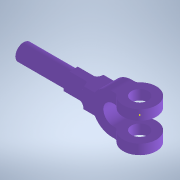
# Autodesk Inventor part: Fork end
Saved by Autodesk Inventor 2021 (Build 250183000, 183)
## iProperties
Created: 2020-01-29
Part Number: Fork end
Material: Plástico PC/ABS
Document SubType Name: Modeling
Designer: aidan
Density: 0.357273 g/cm^3
Appearance: Suave - Blanco
Author: aidan
Autodesk Inventor part; units mm, degrees
ref_plane "YZ Plane" through (0, 0, 0) normal (1, 0, 0) x (0, 1, 0)
ref_plane "XZ Plane" through (0, 0, 0) normal (0, 1, 0) x (-1, 0, 0)
ref_plane "XY Plane" through (0, 0, 0) normal (0, 0, 1) x (1, 0, 0)
sketch "Boceto1" plane through (0, 0, 0) normal (0, 0, 1) x (1, 0, 0)
  point P0 (0, 0)
sketch "Boceto2" plane through (0, 0, 0) normal (0, 1, 0) x (-1, 0, 0)
  line L0 (0, 0) -> (104, 0)
  line L1 (250, -30) -> (250, -90)
  line L2 (104, -120) -> (0, -120)
  arc A0 (100, -90) -> (100, -30) centre (100, -60) ccw
  line L3 (250, -60) -> (250, -30)
  arc A1 (155.9615, -30) -> (104, 0) centre (104, -60) ccw
  arc A2 (104, -120) -> (155.9615, -90) centre (104, -60) ccw
  line L4 (0, -120) -> (0, -90)
  line L5 (0, -30) -> (0, 0)
  line L6 (0, -90) -> (100, -90)
  line L7 (155.9615, -90) -> (250, -90)
  line L8 (250, -30) -> (155.9615, -30)
  line L9 (100, -30) -> (0, -30)
  dimension "d2" = 60
  dimension "d3" = 150
  dimension "d4" = 4
  constraints: 20 end point, 7 perpendicular, 6 point on circle, 3 centre point, 3 parallel, 1 horizontal, 1 midpoint, 1 tangent
  measures "d2" diameter of A0
  measures "d3" distance from line of A0.centre L1
  measures "d4" distance of A0.centre A1.centre
extrude "Extrusión1" add sketch "Boceto2" along normal blind 100
sketch "Boceto3" plane through (-104, 0, 0) normal (0, 0, 1) x (1, 0, 0)
  arc A0 (17.3394, 16) -> (17.3394, 84) centre (54, 50) ccw
  line L0 (0, 100) -> (104, 100) projected
  line L1 (104, 0) -> (104, 100) projected
  line L2 (0, 0) -> (104, 0) projected
  circle A1 centre (54, 50) radius 25
  line L3 (-146, 80) -> (8.1742, 80)
  line L4 (8.1742, 20) -> (-146, 20)
  arc A2 (17.3394, 16) -> (8.1742, 20) centre (8.1742, 7.5) ccw
  arc A3 (8.1742, 80) -> (17.3394, 84) centre (8.1742, 92.5) ccw
  line L5 (-146, 80) -> (-146, 20)
  line L6 (-146, 0) -> (-146, 100) projected
  line L7 (-146, 0) -> (-51.9615, 0) projected
  line L8 (-146, 100) -> (-51.9615, 100) projected
  dimension "d7" = 50
  dimension "d9" = 25
  dimension "d10" = 25
  dimension "d11" = 60
  dimension "d12" = 20
  dimension "d13" = 20
  constraints: 7 tangent, 6 end point, 6 point on circle, 4 centre point, 1 coincident, 1 collinear, 1 parallel
  measures "d7" diameter of A1
  measures "d9" diameter of A2
  measures "d10" diameter of A3
  measures "d11" distance between parallel lines of L4 L3
  measures "d12" distance between parallel lines of L7 L4
  measures "d13" distance between parallel lines of L3 L8
extrude "Extrusión2" cut sketch "Boceto3" against normal blind 200 contours A2 L4 L5 L3 A3 A0 keep common part
sketch "Boceto4" plane through (-250, 20, -30) normal (-1, 0, 0) x (0, 0, 1)
  line L0 (-60, 60) -> (0, 60) projected
  line L1 (0, 60) -> (-17.4, 60)
  line L2 (0, 60) -> (0, 42.6)
  line L3 (0, 0) -> (0, 60) projected
  line L4 (0, 42.6) -> (-17.4, 60)
  line L5 (-42.6, 60) -> (-60, 42.6)
  line L6 (-60, 60) -> (-60, 42.6)
  line L7 (-60, 60) -> (-42.6, 60)
  line L8 (-60, 17.4) -> (-42.6, 0)
  line L9 (-60, 0) -> (-42.6, 0)
  line L10 (-60, 0) -> (-60, 17.4)
  line L11 (-17.4, 0) -> (0, 17.4)
  line L12 (0, 0) -> (0, 17.4)
  line L13 (0, 0) -> (-17.4, 0)
  point P0 (30, -20)
  point P1 (-30, 30)
  dimension "d16" = 17.4
  dimension "d17" = 17.4
  dimension "d20" = 360
  constraints: 24 end point, 2 point on line, 25 other
  measures "d16" distance of L0.end L1.end
  measures "d17" distance of L0.end L2.end
extrude "Extrusión3" cut sketch "Boceto4" against normal blind 60
sketch "Boceto6" plane through (-250, 37.4, -30) normal (-1, 0, 0) x (0, 0, 1)
  circle A0 centre (-30, 12.6) radius 25
  line L0 (0, 0) -> (0, 25.2) projected
  line L1 (-17.4, -17.4) -> (-42.6, -17.4) projected
  point P0 (30, -37.4)
  dimension "d24" = 50
  dimension "d25" = 30
  dimension "d26" = 30
  constraints: 1 centre point
  measures "d24" diameter of A0
  measures "d25" distance from line of A0.centre L0
  measures "d26" distance from line of A0.centre L1
fillet "Empalme1" radius 12 4 edges at (-190, 71.3, -38.7) (-190, 71.3, -81.3) (-190, 28.7, -81.3) (-190, 28.7, -38.7)
extrude "Extrusión4" add sketch "Boceto6" along normal blind 150.7
